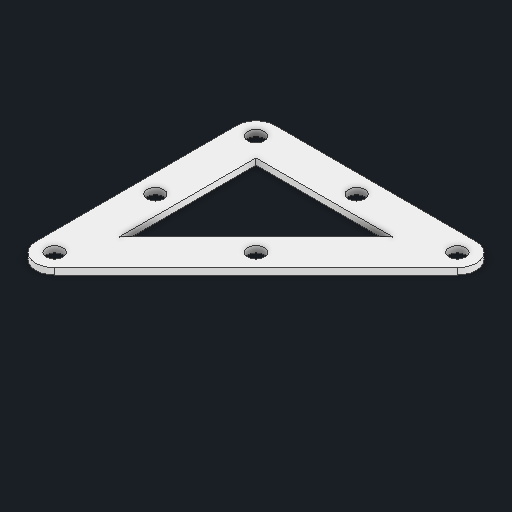
# Autodesk Inventor part: Arm Triangle Gusset
Saved by Autodesk Inventor 2025.1 (Build 291241000, 241)
## iProperties
Created: 2024-10-21
Part Number: Arm Triangle Gusset
Material: Acetal Resin, White
Document SubType Name: Sheet Metal
Designer: averey
Density: 1.425 g/cm^3
Appearance: Smooth - White
Flat Pattern Width: 6.0325 cm
Flat Pattern Length: 6.0325 cm
Flat Pattern Area: 36.3911 cm^2
Sheet Metal Rule: Default_mm
Sheet Metal Width: 2.375 in
Sheet Metal Length: 2.375 in
Sheet Metal Area: 5.641 in^2
Mass: 4.18559 g
Surface Area: 41.3629 cm^2
Volume: 2.93725 cm^3
Author: averey
Autodesk Inventor part; units mm, degrees
ref_plane "YZ Plane" through (0, 0, 0) normal (1, 0, 0) x (0, 1, 0)
ref_plane "XZ Plane" through (0, 0, 0) normal (0, 1, 0) x (-1, 0, 0)
ref_plane "XY Plane" through (0, 0, 0) normal (0, 0, 1) x (1, 0, 0)
sketch "main" plane through (0, 0, 0) normal (0, 0, 1) x (1, 0, 0)
  circle A0 centre (27.8145, 23.5161) radius 2.0955
  circle A1 centre (27.8145, -27.2839) radius 2.0955
  circle A2 centre (-22.9855, -27.2839) radius 2.0955
  arc A3 (-26.3531, -23.9163) -> (-22.9855, -32.0464) centre (-22.9855, -27.2839) ccw
  arc A4 (27.8145, -32.0464) -> (32.577, -27.2839) centre (27.8145, -27.2839) ccw
  arc A5 (32.577, 23.5161) -> (24.4469, 26.8837) centre (27.8145, 23.5161) ccw
  line L0 (32.577, 23.5161) -> (32.577, -27.2839)
  line L1 (27.8145, -32.0464) -> (-22.9855, -32.0464)
  line L2 (24.4469, 26.8837) -> (-26.3531, -23.9163)
  line L3 (-11.4879, -22.5214) -> (23.052, -22.5214)
  line L4 (23.052, -22.5214) -> (23.052, 12.0184)
  line L5 (23.052, 12.0184) -> (-11.4879, -22.5214)
  circle A6 centre (2.4145, -1.8839) radius 2.0955
  point P0 (11.2944, -10.7639)
  dimension "d3" = 4.191
  dimension "d4" = 4.191
  dimension "d5" = 4.191
  dimension "d7" = 9.525
  dimension "d8" = 4.191
  dimension "d9" = 4.7625
  dimension "d10" = 4.7625
  dimension "d11" = 4.7625
  measures "d3" diameter of A1
  measures "d4" diameter of A0
  measures "d5" diameter of A2
  measures "d7" distance between parallel lines of L2 L5
  measures "d8" diameter of A6
  measures "d9" radius of A4
  measures "d10" radius of A5
  measures "d11" radius of A3
sketch "Sketch1" plane through (0, 0, 0) normal (0, 1, 0) x (-1, 0, 0)
  circle A0 centre (-25.4, 0) radius 2.0955
  circle A1 centre (0, 25.4) radius 2.0955
  circle A2 centre (0, 50.8) radius 2.0955
  circle A3 centre (0, 0) radius 2.0955
  circle A4 centre (-50.8, 0) radius 2.0955
  arc A5 (-54.1676, 3.3676) -> (-50.8, -4.7625) centre (-50.8, 0) ccw
  arc A6 (0, -4.7625) -> (4.7625, 0) centre (0, 0) ccw
  arc A7 (4.7625, 50.8) -> (-3.3676, 54.1676) centre (0, 50.8) ccw
  line L0 (4.7625, 50.8) -> (4.7625, 0)
  line L1 (0, -4.7625) -> (-50.8, -4.7625)
  line L2 (-3.3676, 54.1676) -> (-54.1676, 3.3676)
  line L3 (-39.3023, 4.7625) -> (-4.7625, 4.7625)
  line L4 (-4.7625, 4.7625) -> (-4.7625, 39.3023)
  line L5 (-4.7625, 39.3023) -> (-39.3023, 4.7625)
  circle A8 centre (-25.4, 25.4) radius 2.0955
  dimension "d2" = 4.191
  dimension "d6" = 4.191
  constraints: 2 centre point, 1 other
  measures "d2" diameter of A0
  measures "d6" diameter of A1
extrude "Extrusion1" add sketch "Sketch1" along normal blind 1.5875
equation "\"BendRadius\" = Thickness"
equation "\"BendReliefWidth\" = Thickness"
equation "\"BendReliefDepth\" = 0.5 * Thickness"
equation "\"CornerReliefSize\" = 4 * Thickness"
equation "\"MinimumRemnant\" = 2 * Thickness"
equation "\"TransitionRadius\" = BendRadius"
equation "\"JacobiRadiusSize\" = BendRadius"
equation "\"GapSize\" = Thickness"
equation "\"Thickness\" = 1.5875"
body "Solid1"
